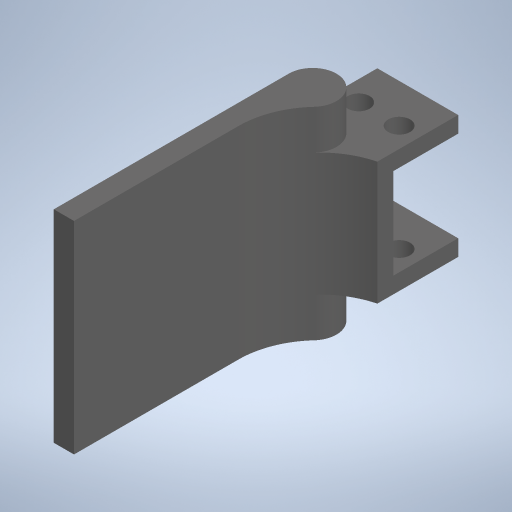
# Autodesk Inventor part: hand_finger
Saved by Autodesk Inventor 2024.1 (Build 281209000, 209)
## iProperties
Created: 2025-02-23
Part Number: hand_finger
Material: 一般
Document SubType Name: Modeling
Designer: hibik
Density: 1 g/cm^3
Appearance: 既定
Author: hibik
Autodesk Inventor part; units mm, degrees
ref_plane "YZ Plane" through (0, 0, 0) normal (1, 0, 0) x (0, 1, 0)
ref_plane "XZ Plane" through (0, 0, 0) normal (0, 1, 0) x (-1, 0, 0)
ref_plane "XY Plane" through (0, 0, 0) normal (0, 0, 1) x (1, 0, 0)
sketch "スケッチ1" plane through (0, 0, 0) normal (1, 0, 0) x (0, 1, 0)
  line L0 (5.6, 0) -> (-5.6, 0)
  line L1 (-5.6, 0) -> (-5.6, -8)
  line L2 (-5.6, -8) -> (5.6, -8)
  line L3 (5.6, -8) -> (5.6, 0)
  line L4 (7.6, -8) -> (-7.6, -8)
  line L5 (-7.6, -8) -> (-7.6, 32)
  line L6 (-7.6, 32) -> (7.6, 32)
  line L7 (7.6, 32) -> (7.6, -8)
  point P0 (0, 0)
  point P1 (0, -8)
  dimension "d0" = 11.2
  dimension "d1" = 8
  dimension "d2" = 15.2
  dimension "d3" = 40
  constraints: 16 end point, 4 parallel, 3 midpoint, 2 horizontal, 2 perpendicular, 1 collinear, 1 vertical alignment
  measures "d0" distance of L1.end L2.end
  measures "d1" distance of L2.end L0.start
  measures "d2" distance of L4.start L4.end
  measures "d3" distance of L6.end L4.start
extrude "押し出し1" add sketch "スケッチ1" along normal blind 10 contours L0 L1 L4 L5 L6 L7 L3
sketch "スケッチ2" plane through (0, 7.6, 32) normal (0, 1, 0) x (1, 0, 0)
  circle A0 centre (2.5, 35.2) radius 1.35
  circle A1 centre (7.5, 35.2) radius 1.35
  line L0 (0, 40) -> (0, 0) projected
  line L1 (10, 40) -> (10, 0) projected
  line L2 (0, 32) -> (10, 32) projected
  dimension "d6" = 2.7
  dimension "d7" = 2.7
  dimension "d8" = 2.5
  dimension "d9" = 2.5
  dimension "d10" = 3.2
  constraints: 2 centre point, 1 horizontal alignment
  measures "d6" diameter of A0
  measures "d7" diameter of A1
  measures "d8" distance from line of L0 A0.centre
  measures "d9" distance from line of L1 A1.centre
  measures "d10" distance from line of L2 A0.centre
extrude "押し出し2" cut sketch "スケッチ2" against normal through all
sketch "スケッチ3" plane through (0, 7.6, 32) normal (0, 1, 0) x (1, 0, 0)
  line L0 (10, 0) -> (2.5, 0)
  line L1 (2.5, 0) -> (2.5, 30)
  line L2 (2.5, 30) -> (10, 30)
  line L3 (10, 30) -> (10, 0)
  line L4 (0, 40) -> (0, 0) projected
  point P0 (0, 32)
  dimension "d13" = 2.5
  dimension "d14" = 30
  constraints: 8 end point, 2 parallel, 1 coincident, 1 horizontal, 1 perpendicular
  measures "d13" distance between parallel lines of L4 L1
  measures "d14" distance of L2.end L0.start
extrude "押し出し3" cut sketch "スケッチ3" against normal through all
fillet "フィレット1" radius 10 1 edges at (2.5, 0, 2)
sketch "スケッチ4" plane through (0, 0, 0) normal (0, 1, 0) x (-1, 0, 0)
  line L0 (0, -8) -> (-10, -8) projected
  line L1 (0, -8) -> (0, 32) projected
  line L2 (0, 32) -> (-2.5, 32) projected
  line L3 (-2.5, 32) -> (-2.5, 11.6825) projected
  circle A0 centre (-2.5, -3.2) radius 1.35 projected
  circle A1 centre (-2.9461, 2.9461) radius 2.9461
  line L4 (0, 0) -> (-10, 0) projected
  line L5 (-10, -8) -> (-10, 2) projected
  arc A2 (-10, 2) -> (-2.5, 11.6825) centre (-12.5, 11.6825) ccw projected
  point P0 (0, 2.9461)
  point P1 (-2.5, 5.8582)
  point P2 (-2.5, 0.034)
  point P3 (-5.1202, 4.9342)
  constraints: 2 tangent, 1 centre point
extrude "押し出し4" add sketch "スケッチ4" along normal mid plane 25 contours A1 A2 L3 L2 L1 | A1
